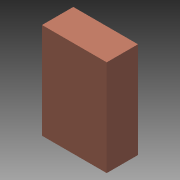
# Autodesk Inventor part: SATA_PLUG
Saved by Autodesk Inventor 2015 SP1 (Build 190203100, 203)
## iProperties
Created: 2015-06-25
Part Number: SATA_PLUG
Material: Generic
Document SubType Name: Modeling
Designer: Patrick
Density: 1 g/cm^3
Appearance: SATA_PLUG, SATA_PLUG
Author: Patrick
Autodesk Inventor part; units mm, degrees
ref_plane "YZ Plane" through (0, 0, 0) normal (1, 0, 0) x (0, 1, 0)
ref_plane "XZ Plane" through (0, 0, 0) normal (0, 1, 0) x (-1, 0, 0)
ref_plane "XY Plane" through (0, 0, 0) normal (0, 0, 1) x (1, 0, 0)
sketch "SATA_PLUG, SATA_PLUG_55" plane through (0, 0, 0) normal (0, 0, 1) x (1, 0, 0)
  line L0 (-6.05, -8.97) -> (-6.05, 8.97)
  line L1 (-6.05, 8.97) -> (6.05, 8.97)
  line L2 (6.05, 8.97) -> (6.05, -8.97)
  line L3 (6.05, -8.97) -> (-6.05, -8.97)
  constraints: 8 end point
extrude "Extrusion1" add sketch "SATA_PLUG, SATA_PLUG_55" along normal blind 5.85
body "Solid1"
